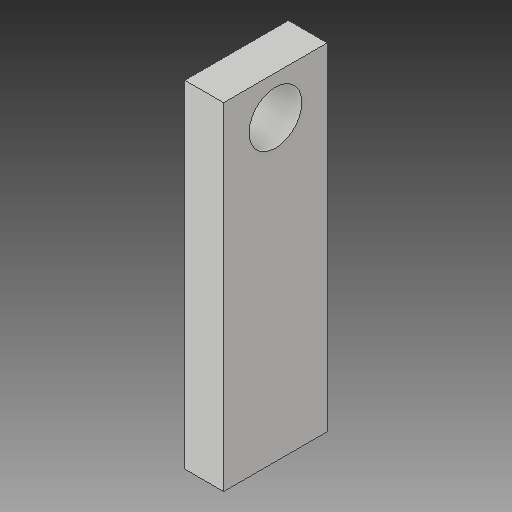
# Autodesk Inventor part: SlidesPivotBracket
Saved by Autodesk Inventor 2019 (Build 230136000, 136)
## iProperties
Created: 2018-11-01
Part Number: SlidesPivotBracket
Material: Generic
Document SubType Name: Modeling
Designer: User
Density: 1 g/cm^3
Appearance: Default
Author: User
Autodesk Inventor part; units mm, degrees
ref_plane "YZ Plane" through (0, 0, 0) normal (1, 0, 0) x (0, 1, 0)
ref_plane "XZ Plane" through (0, 0, 0) normal (0, 1, 0) x (-1, 0, 0)
ref_plane "XY Plane" through (0, 0, 0) normal (0, 0, 1) x (1, 0, 0)
sketch "Sketch1" plane through (0, 0, 0) normal (1, 0, 0) x (0, 1, 0)
  line L0 (0, 0) -> (82.55, 0)
  line L1 (82.55, 0) -> (82.55, -25.4)
  line L2 (82.55, -25.4) -> (0, -25.4)
  line L3 (0, -25.4) -> (0, 0)
  circle A0 centre (73.025, -12.7) radius 6.477
  dimension "d0" = 82.55
  dimension "d1" = 25.4
  dimension "d2" = 12.954
  dimension "d3" = 73.025
  constraints: 8 end point, 2 parallel, 1 centre point, 1 horizontal, 1 perpendicular
  measures "d0" distance of L1.end L2.end
  measures "d1" distance of L0.end L1.end
  measures "d2" diameter of A0
  measures "d3" distance from line of L3 A0.centre
extrude "Extrusion1" add sketch "Sketch1" along normal blind 9.525
sketch "Sketch2" plane through (0, 0, -25.4) normal (0, -1, 0) x (1, 0, 0)
  line L0 (0, 0) -> (0, 25.4) projected
  line L1 (0, 0) -> (9.525, 0) projected
  line L2 (9.525, 25.4) -> (9.525, 0) projected
  line L3 (0, 25.4) -> (9.525, 25.4) projected
  point P0 (4.7625, 22.225)
  point P1 (4.7625, 3.175)
  dimension "d6" = 25.4
  dimension "d7" = 3.175
  dimension "d8" = 3.175
  measures "d6" distance of L2.start L1.end
  measures "d7" distance from line of L3 point (4.763, 22.225)
  measures "d8" distance from line of L1 point (4.763, 3.175)
hole "Hole1" at (4.7625, 0, -3.175) at (4.7625, 0, -22.225) direction (0, 1, 0) diameter 2.6416 depth 25.4 tip angle 118 thread size "6-32 UNC" class "2B" standard "ANSI Unified Screw Threads"
equation "\"d8\" = d7"
body "Solid1"
